load_shaft_8mm (Autodesk Fusion 360 design; units mm, degrees)
part number: 2026-08-30-02-17-07-700
Autodesk Fusion 360 part; units mm, degrees
sketch "Sketch1" plane through (0, 0, 0) normal (0, 1, 0) x (1, 0, 0)
  circle A0 centre (0, 0) radius 4
  dimension "d1" = 8
  constraint coincident A0.centre origin
  measures "d1" diameter of A0
extrude "Extrude1" add sketch "Sketch1" along normal blind 200
sketch "Sketch2" plane through (0, 0, 0) normal (1, 0, 0) x (0, 0, -1)
  circle A0 centre (0, 4.5) radius 1.245
  circle A1 centre (0, 9.5) radius 1.245
  line L0 (4, 0) -> (-4, 0)
  line L1 (0, 0) -> (0, 13) construction
  dimension "d4" = 2.49
  dimension "d5" = 5
  dimension "d6" = 4.5
  constraint equal A0 A1
  constraint coincident L1.start origin
  constraint perpendicular L0 L1
  constraint coincident A0.centre L1
  constraint coincident A1.centre L1
  measures "d4" diameter of A0
  measures "d5" distance of A0.centre A1.centre
  measures "d6" distance of A0.centre L0
extrude "Extrude2" cut sketch "Sketch2" along normal through all and the other way through all
